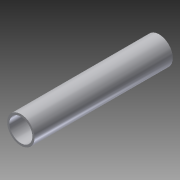
# Autodesk Inventor part: Generic 1ft Segment
Saved by Autodesk Inventor 2015 (Build 190159000, 159)
## iProperties
Created: 2015-04-29
Part Number: Generic 1ft Segment
Material: PVC-Piping
Document SubType Name: Modeling
Designer: 1750019
Density: 1.4 g/cm^3
Appearance: Smooth - White
Mass: 354.74 g
Surface Area: 1080.71 cm^2
Volume: 253.385 cm^3
Author: 1750019
Autodesk Inventor part; units mm, degrees
ref_plane "YZ Plane" through (0, 0, 0) normal (1, 0, 0) x (0, 1, 0)
ref_plane "XZ Plane" through (0, 0, 0) normal (0, 1, 0) x (-1, 0, 0)
ref_plane "XY Plane" through (0, 0, 0) normal (0, 0, 1) x (1, 0, 0)
sketch "Sketch1" plane through (0, 0, 0) normal (0, 0, 1) x (1, 0, 0)
  circle A0 centre (0, 0) radius 25.4
  circle A1 centre (0, 0) radius 30.1625
  dimension "d0" = 50.8
  dimension "d1" = 60.325
  constraints: 2 centre point, 2 coincident
  measures "d0" diameter of A0
  measures "d1" diameter of A1
extrude "Extrusion1" add sketch "Sketch1" along normal blind 304.8
body "Solid1"
